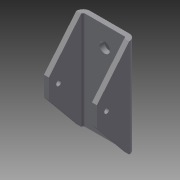
# Autodesk Inventor part: BackPistonHinge-Tower
Saved by Autodesk Inventor 2013 (Build 170138000, 138)
## iProperties
Created: 2013-02-07
Part Number: BackPistonHinge-Tower
Material: Generic
Document SubType Name: Sheet Metal
Designer: motoennies
Density: 1 g/cm^3
Sheet Metal Rule: Default
Author: motoennies
Autodesk Inventor part; units mm, degrees
ref_plane "YZ Plane" through (0, 0, 0) normal (1, 0, 0) x (0, 1, 0)
ref_plane "XZ Plane" through (0, 0, 0) normal (0, 1, 0) x (-1, 0, 0)
ref_plane "XY Plane" through (0, 0, 0) normal (0, 0, 1) x (1, 0, 0)
sketch "Sketch1" plane through (0, 0, 0) normal (0, 0, 1) x (1, 0, 0)
  line L0 (0, 0) -> (25.4, 0)
  line L1 (25.4, 0) -> (25.4, 63.5)
  line L2 (25.4, 63.5) -> (0, 63.5)
  line L3 (0, 63.5) -> (0, 0)
  circle A0 centre (12.7, 50.8) radius 3.3782
  circle A1 centre (12.7, 12.7) radius 3.3782
  dimension "d0" = 25.4
  dimension "d1" = 63.5
  dimension "d2" = 6.7564
  dimension "d3" = 6.7564
  dimension "d4" = 12.7
  dimension "d5" = 12.7
  dimension "d6" = 12.7
  dimension "d7" = 12.7
  measures "d0" distance of L0.start L0.end
  measures "d1" distance of L0.end L1.end
  measures "d2" diameter of A0
  measures "d3" diameter of A1
  measures "d4" distance from line of L0 A1.centre
  measures "d5" distance from line of L1 A1.centre
  measures "d6" distance from line of L2 A0.centre
  measures "d7" distance from line of L1 A0.centre
extrude "Plate1" add sketch "Sketch1" along normal blind 3.175
sketch "Sketch2" plane through (26.67, 63.5, 4.445) normal (1, 0, 0) x (0, 1, 0)
  line L0 (-63.5, 0) -> (0, 0)
  line L1 (0, 0) -> (0, 20.955)
  line L2 (0, 20.955) -> (-63.5, 20.955)
  line L3 (-63.5, 20.955) -> (-63.5, 0)
  constraints: 6 end point, 1 horizontal, 1 perpendicular, 1 vertical
edge flange "Flange1" height 25.4 angle 90 thickness 3.175 bend radius 1.27 thickness toward (1, 0, 0) relief tear relief width 3.175 relief depth 1.5875 edges at (25.4, 31.75, 3.175) wall of the first edge with corners at (26.67, 0, 4.445) (26.67, 63.5, 4.445) (26.67, 63.5, 25.4) (26.67, 0, 25.4)
bend "Bend1"
corner "Corner1"
sketch "Sketch3" plane through (29.845, 0, 25.4) normal (1, 0, 0) x (0, 0, -1)
  line L0 (0, 63.5) -> (20.955, 63.5) projected
  line L1 (0, 0) -> (0, 63.5) projected
  line L2 (20.955, 0) -> (0, 0) projected
  circle A0 centre (6.35, 31.75) radius 1.5875
  line L3 (0, 38.1) -> (20.955, 63.5)
  line L4 (0, 25.4) -> (20.955, 0)
  point P0 (25.4, 0)
  dimension "d19" = 3.175
  dimension "d20" = 6.35
  dimension "d21" = 31.75
  dimension "d22" = 12.7
  dimension "d23" = 25.4
  constraints: 4 end point, 2 point on line, 1 centre point
  measures "d19" diameter of A0
  measures "d20" distance from line of L1 A0.centre
  measures "d21" distance from line of L2 A0.centre
  measures "d22" distance of L3.start L4.start
  measures "d23" distance from line of L2 L4.start
sketch "Sketch4" plane through (-1.27, 0, 4.445) normal (-1, 0, 0) x (0, -1, 0)
  line L0 (-63.5, 0) -> (0, 0)
  line L1 (0, 0) -> (0, 20.955)
  line L2 (0, 20.955) -> (-63.5, 20.955)
  line L3 (-63.5, 20.955) -> (-63.5, 0)
  constraints: 6 end point, 1 horizontal, 1 perpendicular, 1 vertical
edge flange "Flange2" height 25.4 angle 90 thickness 3.175 bend radius 1.27 thickness toward (-1, 0, 0) relief tear relief width 3.175 relief depth 1.5875 edges at (0, 31.75, 3.175) wall of the first edge with corners at (-1.27, 63.5, 4.445) (-1.27, 0, 4.445) (-1.27, 0, 25.4) (-1.27, 63.5, 25.4)
bend "Bend2"
corner "Corner2"
extrude "Extrusion1" cut sketch "Sketch3" against normal blind 76.2
equation "\"d9\" = BendReliefWidth"
equation "\"d10\" = BendReliefDepth"
equation "\"d11\" = MinimumRemnant"
equation "\"d12\" = BendRadius"
equation "\"d16\" = CornerReliefSize"
equation "\"d17\" = GapSize"
equation "\"d18\" = JacobiRadiusSize"
equation "\"d26\" = BendReliefWidth"
equation "\"d27\" = BendReliefDepth"
equation "\"d28\" = MinimumRemnant"
equation "\"d29\" = BendRadius"
equation "\"d33\" = CornerReliefSize"
equation "\"d34\" = GapSize"
equation "\"d35\" = JacobiRadiusSize"
equation "\"BendRadius\" = Thickness"
equation "\"BendReliefWidth\" = Thickness"
equation "\"BendReliefDepth\" = 0.5 * Thickness"
equation "\"CornerReliefSize\" = 4 * Thickness"
equation "\"MinimumRemnant\" = 2 * Thickness"
equation "\"TransitionRadius\" = BendRadius"
equation "\"JacobiRadiusSize\" = BendRadius"
equation "\"GapSize\" = Thickness"
equation "\"d8\" = BendRadius"
equation "\"Thickness\" = 3.175"
body "Solid1"
